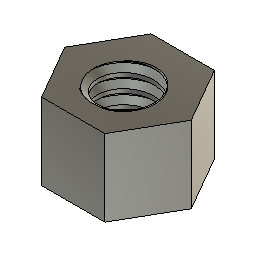
tripod_bolt (Autodesk Fusion 360 design; units mm, degrees)
Autodesk Fusion 360 part; units mm, degrees
cylinder "CylinderPrimitive1" add diameter 6.35 height 20 placed x (1, 0, 0) y (0, 1, 0) z (0, 0, 1) at (0, 0, 0) makes body 1 in component "thread"
thread "Thread1" "ANSI Unified Screw Threads 0.25 1/4-20 UNC 3A" major diameter 6.2484 minor diameter 4.8387 pitch 1.27 angle 60 modelled right hand crest width 0.1965 on face at (3.1592, -0.3161, 13.3333) crest through (3.1242, 0, -0.3175) on bodies 1 in component "thread"
sketch "Sketch3" plane through (0, 0, 0) normal (0, 0, 1) x (1, 0, 0) in component "nut"
  circle A0 centre (0, 0) radius 5
  circle A1 centre (0, 0) radius 3.175
  line L0 (5.7735, 0) -> (2.8868, 5)
  line L1 (2.8868, 5) -> (-2.8868, 5)
  line L2 (-2.8868, 5) -> (-5.7735, 0)
  line L3 (-5.7735, 0) -> (-2.8868, -5)
  line L4 (-2.8868, -5) -> (2.8868, -5)
  line L5 (2.8868, -5) -> (5.7735, 0)
  dimension "d7" = 10
  dimension "d8" = 6.35
  constraint coincident A0.centre A1.centre
  constraint horizontal L4
  measures "d7" diameter of A0
  measures "d8" diameter of A1
extrude "Extrude2" add sketch "Sketch3" along normal blind 7 separate body makes body 2 in component "nut"
thread "Thread1'" "ANSI Unified Screw Threads 0.25 1/4-20 UNC 3B" major diameter 6.35 minor diameter 5.1156 pitch 1.27 angle 60 modelled right hand crest width 0.3725 on face at (3.1711, -0.1583, 2.3333) crest through (2.5578, 0, 0.3175) on bodies 2 in component "nut"
move_face "OffsetFaces1" [suppressed] in component "nut"
move_face "OffsetFaces2" [suppressed] in component "nut"
component "thread" placed x (1, 0, 0) y (0, 1, 0) z (0, 0, 1) at (0, 0, 0)
component "nut" placed x (1, 0, 0) y (0, 1, 0) z (0, 0, 1) at (0, 0, 0)
named bodies: "nut"
